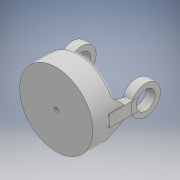
# Autodesk Inventor part: Wrist2
Saved by Autodesk Inventor 2017 (Build 210142000, 142)
## iProperties
Created: 2016-12-26
Part Number: Wrist2
Material: Generic
Document SubType Name: Modeling
Designer: Samanth
Density: 1 g/cm^3
Appearance: Default
Author: Samanth
Autodesk Inventor part; units mm, degrees
ref_plane "YZ Plane" through (0, 0, 0) normal (1, 0, 0) x (0, 1, 0)
ref_plane "XZ Plane" through (0, 0, 0) normal (0, 1, 0) x (-1, 0, 0)
ref_plane "XY Plane" through (0, 0, 0) normal (0, 0, 1) x (1, 0, 0)
sketch "Sketch1" plane through (0, 0, 0) normal (0, 0, 1) x (1, 0, 0)
  line L0 (0, 0) -> (60, 0)
  line L1 (60, 0) -> (60, 30)
  line L2 (0, 30) -> (0, 0)
  line L3 (75, 0) -> (75, -15)
  line L4 (75, -15) -> (60, -15)
  line L5 (0, 30) -> (-15, 30)
  line L6 (75, 30) -> (75, -15)
  line L7 (75, -15) -> (-15, -15)
  line L8 (-15, -15) -> (-15, 30)
  line L9 (60, 30) -> (75, 30)
  constraints: 20 end point, 3 perpendicular, 1 horizontal, 1 parallel
extrude "Extrusion1" add sketch "Sketch1" along normal blind 15
sketch "Sketch2" plane through (75, -15, 0) normal (1, 0, 0) x (0, 0, -1)
  line L0 (0, 45) -> (-15, 45) projected
  circle A0 centre (-7.5, 45) radius 4.4
  point P0 (0, 15)
  dimension "d9" = 8.8
  constraints: 1 centre point, 1 midpoint
  measures "d9" diameter of A0
extrude "Extrusion2" cut sketch "Sketch2" against normal blind 105
sketch "Sketch3" plane through (0, 0, 15) normal (0, 0, 1) x (1, 0, 0)
  line L0 (-15, 30) -> (0, 30) projected
  line L1 (0, 30) -> (0, 0) projected
  arc A0 (-7.5, 30) -> (0, 0) centre (50.5521, 28.5755) ccw
  line L2 (60, 30) -> (60, 0) projected
  line L3 (75, 30) -> (60, 30) projected
  arc A1 (60, 0) -> (67.5, 30) centre (29.1821, 23.642) ccw
  line L4 (0, 0) -> (0, 30)
  line L5 (-7.5, 30) -> (0, 30)
  line L6 (67.5, 30) -> (60, 30)
  line L7 (60, 30) -> (60, 0)
  constraints: 8 end point, 4 point on circle, 2 centre point, 2 collinear, 2 midpoint, 2 perpendicular
extrude "Extrusion3" cut sketch "Sketch3" against normal blind 105
sketch "Sketch4" plane through (0, 0, 0) normal (0, 1, 0) x (1, 0, 0)
  line L0 (0, 0) -> (0, -15) projected
  line L1 (0, -7.5) -> (30, 0)
  line L2 (0, 0) -> (60, 0) projected
  line L3 (30, -7.5) -> (30, 0)
  circle A0 centre (30, -7.5) radius 2.5
  dimension "d14" = 5
  constraints: 4 end point, 2 midpoint, 1 centre point, 1 coincident, 1 perpendicular
  measures "d14" diameter of A0
extrude "Extrusion4" cut sketch "Sketch4" against normal blind 20 contours A0
sketch "Sketch5" plane through (-15, -15, 0) normal (0, -1, 0) x (1, 0, 0)
  circle A0 centre (45, 7.5) radius 2.5 projected
  circle A1 centre (45, 7.5) radius 2.5
  circle A2 centre (45, 7.5) radius 45
  point P0 (15, 0)
  constraints: 2 centre point, 2 coincident
extrude "Extrusion5" add sketch "Sketch5" along normal blind 20 and the other way blind 10
chamfer "Chamfer1" distance 9 angle 45 2 edges at (30, -5, 15) (30, -5, 0)
sketch "Sketch6" plane through (75, -15, 0) normal (1, 0, 0) x (0, 0, -1)
  arc A0 (-11.9, 45) -> (-3.1, 45) centre (-7.5, 45) ccw projected
  circle A1 centre (-7.5, 45) radius 11.5
  circle A2 centre (-7.5, 45) radius 18
  point P0 (0, 15)
  dimension "d24" = 23
  dimension "d25" = 36
  constraints: 2 centre point, 2 coincident
  measures "d24" diameter of A1
  measures "d25" diameter of A2
extrude "Extrusion6" add sketch "Sketch6" against normal blind 11 separate body
sketch "Sketch7" plane through (-15, -15, 0) normal (-1, 0, 0) x (0, 0, 1)
  arc A0 (3.1, 45) -> (11.9, 45) centre (7.5, 45) ccw projected
  circle A1 centre (7.5, 45) radius 18
  circle A2 centre (7.5, 45) radius 11.5
  point P0 (0, 15)
  constraints: 2 centre point, 2 coincident
extrude "Extrusion7" add sketch "Sketch7" against normal blind 11 separate body
sketch "Sketch8" plane through (75, 30, 7.5) normal (1, 0, 0) x (0, 0, -1)
  circle A0 centre (0, 0) radius 11.5347
  point P0 (7.5, -30)
  constraints: 1 centre point
extrude "Extrusion8" cut sketch "Sketch8" against normal blind 96.75 bodies 2 1
fillet "Fillet1" radius 3 2 edges at (30, -5, -37.5) (30, -5, 52.5)
body "Solid1"
body "Solid2"
body "Solid3"
